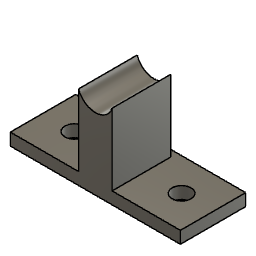
Led_Cover (Autodesk Fusion 360 design; units mm, degrees)
Autodesk Fusion 360 part; units mm, degrees
sketch "Sketch1" plane through (0, 0, 0) normal (0, 1, 0) x (1, 0, 0)
  line L0 (2.5, -4.375) -> (-2.5, -4.375)
  line L1 (-2.5, -4.375) -> (-2.5, 4.375)
  line L2 (-2.5, 4.375) -> (2.5, 4.375)
  line L3 (2.5, 4.375) -> (2.5, -4.375)
  line L4 (0, -17.6215) -> (0, 10.113) construction
  line L5 (14.6118, 0) -> (-14.9327, 0) construction
  dimension "d1" = 5
  dimension "d2" = 8.75
  constraint horizontal L0
  constraint vertical L1
  constraint horizontal L2
  constraint vertical L3
  constraint parallel L1 L4
  constraint perpendicular L3 L5
  constraint coincident origin L5
  constraint coincident origin L4
  constraint symmetric L1 L3 L4
  constraint symmetric L0 L2 L5
  measures "d1" distance of L0.start L0.end
  measures "d2" distance of L0.end L1.end
extrude "Extrude1" add sketch "Sketch1" along normal blind 8.875
sketch "Sketch2" plane through (0, 0, 4.375) normal (0, 0, 1) x (1, 0, 0)
  line L0 (-2.5, 0) -> (2.5, 0)
  line L1 (2.5, 0) -> (2.5, 8.875)
  line L2 (2.5, 8.875) -> (-2.5, 8.875)
  line L3 (-2.5, 8.875) -> (-2.5, 0)
  line L4 (-2.5, 8.875) -> (2.5, 8.875)
  line L5 (2.5, 8.875) -> (2.5, 11.5)
  line L6 (2.5, 11.5) -> (-2.5, 11.5)
  line L7 (-2.5, 11.5) -> (-2.5, 8.875)
  circle A0 centre (0, 11.5) radius 2.625
  line L8 (0, 0) -> (0, 8.875) construction
  dimension "d10" = 5.25
  constraint horizontal L4
  constraint vertical L5
  constraint horizontal L6
  constraint vertical L7
  constraint coincident L2.end L3.start
  constraint tangent L4 A0
  constraint coincident L8.start origin
  constraint midpoint L4 L8.end
  constraint perpendicular L4 L8
  constraint coincident A0.centre L8
  constraint coincident L6 A0.centre
  measures "d10" diameter of A0
extrude "Extrude3" add sketch "Sketch2" against normal blind 8.75 contours L2 L4 L7 A0 | L2 L4 L5 A0
sketch "Sketch3" plane through (0, 0, 0) normal (0, -1, 0) x (1, 0, 0)
  line L0 (-2.5, -4.375) -> (2.5, -4.375)
  line L1 (2.5, -4.375) -> (2.5, 4.375)
  line L2 (2.5, 4.375) -> (-2.5, 4.375)
  line L3 (-2.5, 4.375) -> (-2.5, -4.375)
  line L4 (-12.7, 4.375) -> (12.7, 4.375)
  line L5 (12.7, 4.375) -> (12.7, -5.375)
  line L6 (12.7, -5.375) -> (-12.7, -5.375)
  line L7 (-12.7, -5.375) -> (-12.7, 4.375)
  line L8 (0, 4.375) -> (0, -4.375) construction
  line L9 (12.7, -0.5) -> (-12.7, -0.5) construction
  circle A0 centre (-8, -0.5) radius 1.42
  circle A1 centre (8, -0.5) radius 1.42
  dimension "d16" = 25.4
  dimension "d17" = 2.84
  dimension "d18" = 16
  dimension "d21" = 9.75
  dimension "d22" = 4.875
  constraint horizontal L4
  constraint vertical L5
  constraint horizontal L6
  constraint vertical L7
  constraint midpoint L2 L8.start
  constraint midpoint L0 L8.end
  constraint midpoint L4 L8.start
  constraint coincident L9 A0.centre
  constraint coincident L9 A1.centre
  constraint equal A0 A1
  constraint symmetric L8 A0 A1
  measures "d16" distance of L4.start L4.end
  measures "d17" diameter of A0
  measures "d18" distance of A0.centre A1.centre
  measures "d21" distance of L4.start L6.end
  measures "d22" distance of L4 L9
extrude "Extrude5" add sketch "Sketch3" along normal blind 1.8
